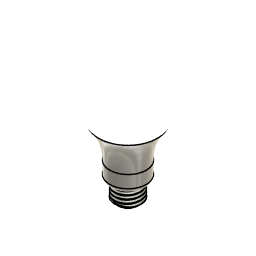
Oct19_Light_Bulb (Autodesk Fusion 360 design; units mm, degrees)
part number: 2025-10-19-23-24-09-821
part number: 2025-10-19-23-24-55-392
Autodesk Fusion 360 part; units mm, degrees
cylinder "CylinderPrimitive1" add diameter 30 height 40 placed x (1, 0, 0) y (0, 1, 0) z (0, 0, 1) at (0, 0, 0) makes body 1 in component "Light Bulb"
sketch "Sketch2" plane through (0, 0, 0) normal (0, 1, 0) x (1, 0, 0) in component "Light Bulb"
  line L0 (-15, -40) -> (15, -40) construction
  line L1 (0, -40) -> (0, -60) construction
  point P0 (-15, -40)
  point P1 (15, -40)
  dimension "d4" = 20
  constraint coincident P0 L0.start
  constraint coincident P1 L0.end
  constraint midpoint L0 L1.start
  constraint perpendicular L0 L1
  measures "d4" distance of L1.start L1.end
sphere "SpherePrimitive1" add diameter 61 placed x (1, 0, 0) y (0, 0, -1) z (0, 1, 0) at (0, 0, 60) bodies 1 in component "Light Bulb"
fillet "Fillet1" radius 45 1 edges at (-13.9849, 5.4242, 33.4435) on bodies 1 in component "Light Bulb"
fillet "Fillet1" radius 4 1 edges at (-13.9849, 5.4242, 0) on bodies 1 in component "Light Bulb"
cylinder "CylinderPrimitive2" add diameter 22 height -12 placed x (1, 0, 0) y (0, 1, 0) z (0, 0, 1) at (0, 0, 0) separate body makes body 2 in component "Light Bulb"
cylinder "CylinderPrimitive3" add diameter 22 height 3 placed x (0, 1, 0) y (1, 0, 0) z (0, 0, -1) at (0, 0, -12) separate body makes body 3 in component "Light Bulb"
thread "Thread2" "ANSI Metric M Profile 22.0 M22x3 M22x3 6g" major diameter 21.7645 minor diameter 18.3374 pitch 3 angle 60 modelled right hand crest width 0.4298 on face at (10.9453, -1.0952, -4) crest through (0, 10.8823, 0.75) on bodies 2 in component "Light Bulb"
chamfer "Chamfer1" distance 3 angle 45 1 edges at (-3.9778, -10.2556, -15) on bodies 3 in component "Light Bulb"
fillet "Fillet2" radius 2 1 edges at (-2.8929, 7.4586, -15) on bodies 3 in component "Light Bulb"
cylinder "CylinderPrimitive4" add diameter 14.343 height 2 placed x (0, 1, 0) y (1, 0, 0) z (0, 0, -1) at (0, 0, -15) bodies 3 in component "Light Bulb"
chamfer "Chamfer2" distance 2 angle 45 1 edges at (-2.5933, -6.6862, -17) on bodies 3 in component "Light Bulb"
component "Light Bulb" placed x (1, 0, 0) y (0, 1, 0) z (0, 0, 1) at (0, 0, 0)
